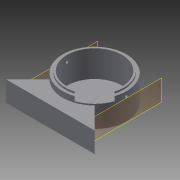
# Autodesk Inventor part: clock_case_bottom
Saved by Autodesk Inventor 2015 SP2 (Build 190223200, 223)
## iProperties
Created: 2016-03-14
Part Number: clock_case_bottom
Material: Generic
Document SubType Name: Modeling
Designer: mca20
Density: 1 g/cm^3
Appearance: Default
Author: mca20
Autodesk Inventor part; units mm, degrees
ref_plane "XZ Plane" through (0, 0, 0) normal (0, 1, 0) x (-1, 0, 0)
ref_plane "XY Plane" through (0, 0, 0) normal (0, 0, 1) x (1, 0, 0)
sketch "Sketch1" plane through (0, 0, 0) normal (0, 1, 0) x (-1, 0, 0)
  circle A0 centre (0, 0) radius 36
  dimension "d0" = 72
  constraints: 1 centre point, 1 coincident
  measures "d0" diameter of A0
extrude "Extrusion1" add sketch "Sketch1" along normal blind 1.5
sketch "Sketch2" plane through (0, 1.5, 0) normal (0, 1, 0) x (1, 0, 0)
  circle A0 centre (0, 0) radius 36 projected
  circle A1 centre (0, 0) radius 33
  circle A2 centre (0, 0) radius 31
  dimension "d3" = 3
  dimension "d4" = 2
  dimension "d23" = 72
  dimension "d24" = 66
  dimension "d25" = 62
  constraints: 2 centre point
  measures "d3" radial gap between concentric circles of A0 A1
  measures "d4" radial gap between concentric circles of A1 A2
  measures "d23" diameter of A0
  measures "d24" diameter of A1
  measures "d25" diameter of A2
extrude "Extrusion2" add sketch "Sketch2" along normal blind 30 contours A1
sketch "Sketch3" plane through (0, 1.5, 0) normal (0, 1, 0) x (1, 0, 0)
  circle A0 centre (0, 0) radius 36 projected
  circle A1 centre (0, 0) radius 33 projected
  dimension "d51" = 72
  dimension "d52" = 66
  measures "d51" diameter of A0
  measures "d52" diameter of A1
extrude "Extrusion3" add sketch "Sketch3" along normal blind 28
sketch "Sketch5" plane through (0, 31.5, 0) normal (0, 1, 0) x (1, 0, 0)
  circle A0 centre (0, 0) radius 22.5
  line L0 (-22.5, 0) -> (7.2195, 0) construction
  line L1 (0, -22.5) -> (23.761, -22.5) construction
  line L2 (22.5, 0) -> (0, -22.5)
  line L3 (0, -22.5) -> (19.2037, -41.7037)
  line L4 (0, -22.5) -> (27.1581, -22.5) construction
  line L5 (22.5, 0) -> (46.5776, -24.0776)
  line L6 (22.5, 0) -> (56.5508, 0) construction
  line L7 (46.5776, -24.0776) -> (19.2037, -41.7037)
  dimension "d13" = 45
  dimension "d18" = 45
  dimension "d19" = 45
  constraints: 16 end point, 4 horizontal, 3 point on circle, 2 equal length, 1 centre point, 1 coincident
  measures "d13" diameter of A0
  measures "d18" angle of L3 L4
  measures "d19" angle of L5 L6
extrude "Extrusion4" cut sketch "Sketch5" against normal blind 7 contours L5 L7 L3 A0 | A0 L2 picked at (12.1762, -13.3637)
ref_plane "Work Plane1" through (-36, 0, 0) normal (1, 0, 0) x (0, 1, 0)
sketch "Sketch7" plane through (-36, 0, 0) normal (1, 0, 0) x (0, 1, 0)
  circle A0 centre (24.5, 0) radius 1.5
  line L0 (29.5, -36) -> (29.5, 36) projected
  point P0 (0, 0)
  point P1 (29.5, 11.585)
  point P2 (29.5, 34.085)
  dimension "d26" = 3
  dimension "d27" = 5
  constraints: 1 centre point
  measures "d26" diameter of A0
  measures "d27" distance from line of L0 A0.centre
hole "Hole1" at (-36, 24.5, 0) direction (1, 0, 0) diameter 3 depth 8 tip angle 118
ref_plane "Work Plane2" through (36, 0, 0) normal (1, 0, 0) x (0, 1, 0)
sketch "Sketch8" plane through (36, 0, 0) normal (1, 0, 0) x (0, 1, 0)
  circle A0 centre (24.5, 0) radius 1.5
  line L0 (29.5, -36) -> (29.5, 36) projected
  point P0 (0, 0)
  point P1 (29.5, 11.585)
  point P2 (29.5, 34.085)
  dimension "d42" = 3
  dimension "d43" = 5
  constraints: 1 centre point
  measures "d42" diameter of A0
  measures "d43" distance from line of L0 A0.centre
hole "Hole2" at (36, 24.5, 0) direction (-1, 0, 0) diameter 3 depth 8 tip angle 118
sketch "Sketch10" plane through (0, 1.5, 0) normal (0, 1, 0) x (1, 0, 0)
  line L0 (0, 0) -> (0, -50)
  line L1 (0, 0) -> (49.9372, -49.9372)
  line L2 (0, 0) -> (70.6219, 0) construction
  line L3 (0, 0) -> (-49.9372, -49.9372)
  line L4 (0, 0) -> (70.6219, 0) construction
  circle A0 centre (0, 0) radius 36 projected
  line L5 (-49.9372, -49.9372) -> (49.9372, -49.9372)
  point P0 (-25.4558, -25.4558)
  point P1 (25.4558, -25.4558)
  dimension "d44" = 50
  dimension "d45" = 45
  dimension "d46" = 135
  constraints: 12 end point, 3 horizontal, 2 equal length, 2 point on circle, 2 point on line, 1 vertical
  measures "d44" distance of L0.start L0.end
  measures "d45" angle of L1 L2
  measures "d46" angle of L3 L4
extrude "Extrusion5" add sketch "Sketch10" along normal blind 21.5 and the other way blind 1.5 contours A0 L1 L5 L0 | L0 L5 L3 A0
body "Solid1"
